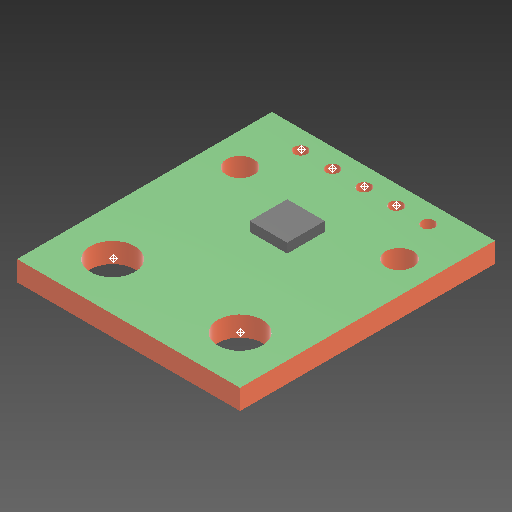
# Autodesk Inventor part: ACS711EX
Saved by Autodesk Inventor 2020.2 (Build 242310000, 310)
## iProperties
Created: 2020-04-10
Part Number: ACS711EX
Material: Phenolic Resin
Document SubType Name: Modeling
Designer: agmlego
Mass: 0.737685 g
Surface Area: 8.73919 cm^2
Volume: 0.534554 cm^3
Density: 1.38 g/cm^3
Appearance: Smooth - Light Orange
GlobalPropertyList: <PropertyList/>
Author: agmlego
Autodesk Inventor part; units mm, degrees
ref_plane "YZ Plane" through (0, 0, 0) normal (1, 0, 0) x (0, 1, 0)
ref_plane "XZ Plane" through (0, 0, 0) normal (0, 1, 0) x (-1, 0, 0)
ref_plane "XY Plane" through (0, 0, 0) normal (0, 0, 1) x (1, 0, 0)
sketch "Sketch1" plane through (0, 0, 0) normal (0, 1, 0) x (-1, 0, 0)
  line L0 (0, 0) -> (17.78, 0)
  line L1 (17.78, 0) -> (17.78, -20.32)
  line L2 (17.78, -20.32) -> (0, -20.32)
  line L3 (0, -20.32) -> (0, 0)
  dimension "d0" = 20.32
  dimension "d1" = 17.78
  constraints: 8 end point, 2 parallel, 1 horizontal, 1 perpendicular
  measures "d0" distance of L0.end L1.end
  measures "d1" distance of L0.start L0.end
extrude "PCB" add sketch "Sketch1" along normal blind 1.6
sketch "Sketch2" plane through (0, 1.6, 0) normal (0, 1, 0) x (1, 0, 0)
  line L0 (0, 20.32) -> (-17.78, 20.32) construction
  line L1 (0, 20.32) -> (-17.78, 20.32) construction
  line L2 (-8.89, 20.32) -> (-8.89, 0) construction
  line L3 (-17.78, 0) -> (0, 0) construction
  line L4 (0, 0) -> (0, 20.32) construction
  point P0 (-3.81, 18.796)
  point P1 (-6.35, 18.796)
  point P2 (-2.54, 15.24)
  point P3 (-3.81, 3.81)
  point P4 (-13.97, 18.796)
  point P5 (-11.43, 18.796)
  point P6 (-15.24, 15.24)
  point P7 (-13.97, 3.81)
  point P8 (-8.89, 18.796)
  dimension "d4" = 1.524
  dimension "d5" = 3.81
  dimension "d6" = 2.54
  dimension "d7" = 2.54
  dimension "d8" = 5.08
  dimension "d9" = 3.81
  dimension "d10" = 16.51
  constraints: 4 symmetric about line, 3 horizontal alignment, 2 end point, 2 midpoint, 1 point on line
  measures "d4" distance from line of L0 point (-3.81, 18.796)
  measures "d5" distance from line of L4 point (-3.81, 18.796)
  measures "d6" distance of point (-6.35, 18.796) point (-3.81, 18.796)
  measures "d7" distance from line of L4 point (-2.54, 15.24)
  measures "d8" distance from line of L0 point (-2.54, 15.24)
  measures "d9" distance from line of L4 point (-3.81, 3.81)
  measures "d10" distance from line of L0 point (-3.81, 3.81)
hole "0.1\" Pin Headers" at (-13.97, 1.6, -18.796) at (-11.43, 1.6, -18.796) at (-8.89, 1.6, -18.796) at (-6.35, 1.6, -18.796) at (-3.81, 1.6, -18.796) direction (0, -1, 0) diameter 1.016 end through all
hole "Mounting" at (-15.24, 1.6, -15.24) at (-2.54, 1.6, -15.24) direction (0, -1, 0) diameter 2.1844 end through all
hole "Current Sense" at (-3.81, 1.6, -3.81) at (-13.97, 1.6, -3.81) direction (0, -1, 0) diameter 3.556 end through all
sketch "Sketch3" plane through (0, 1.6, 0) normal (0, 1, 0) x (1, 0, 0)
  line L0 (-10.39, 11.1478) -> (-7.39, 11.1478)
  line L1 (-7.39, 11.1478) -> (-7.39, 14.1478)
  line L2 (-7.39, 14.1478) -> (-10.39, 14.1478)
  line L3 (-10.39, 14.1478) -> (-10.39, 11.1478)
  line L4 (-8.89, 20.32) -> (-8.89, 0) construction
  circle A0 centre (-15.24, 15.24) radius 1.0922 projected
  point P0 (0, 0)
  point P1 (-8.89, 14.1478)
  dimension "d32" = 3
  constraints: 8 end point, 2 parallel, 2 perpendicular, 1 horizontal, 1 midpoint, 1 point on line, 1 tangent
  measures "d32" distance of L2.end L0.start
extrude "ACS711" add sketch "Sketch3" along normal blind 0.75 contours L3 L2 L1 L0
sketch "Sketch4" plane through (0, 1.6, 0) normal (0, 1, 0) x (1, 0, 0)
  circle A0 centre (-13.97, 18.796) radius 0.508 projected
sketch "Sketch5" plane through (0, 1.6, 0) normal (0, 1, 0) x (1, 0, 0)
  circle A0 centre (-11.43, 18.796) radius 0.508 projected
sketch "Sketch6" plane through (0, 1.6, 0) normal (0, 1, 0) x (1, 0, 0)
  circle A0 centre (-8.89, 18.796) radius 0.508 projected
sketch "Sketch7" plane through (0, 1.6, 0) normal (0, 1, 0) x (1, 0, 0)
  circle A0 centre (-6.35, 18.796) radius 0.508 projected
sketch "Sketch8" plane through (0, 1.6, 0) normal (0, 1, 0) x (1, 0, 0)
  circle A0 centre (-13.97, 3.81) radius 1.778 projected
sketch "Sketch9" plane through (0, 1.6, 0) normal (0, 1, 0) x (1, 0, 0)
  circle A0 centre (-3.81, 3.81) radius 1.778 projected
body "Solid1"
